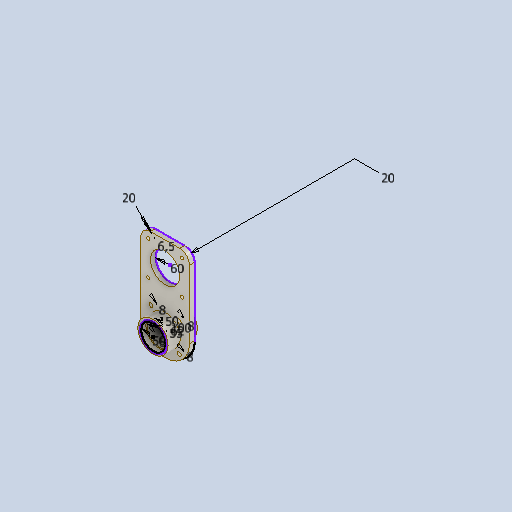
# Autodesk Inventor part: podstwa_obrotowa
Saved by Autodesk Inventor 2023 (Build 270158000, 158)
## iProperties
Created: 2023-03-28
Part Number: podstwa_obrotowa
Material: Tytan
Document SubType Name: Modeling
Designer: krzys
Density: 4.51 g/cm^3
Appearance: Tytan
Mass: 847.85 g
Surface Area: 700.811 cm^2
Volume: 187.993 cm^3
Author: krzys
Autodesk Inventor part; units mm, degrees
ref_plane "YZ Plane" through (0, 0, 0) normal (1, 0, 0) x (0, 1, 0)
ref_plane "XZ Plane" through (0, 0, 0) normal (0, 1, 0) x (-1, 0, 0)
ref_plane "XY Plane" through (0, 0, 0) normal (0, 0, 1) x (1, 0, 0)
sketch "Szkic1" plane through (0, 0, 0) normal (0, 0, 1) x (1, 0, 0)
  circle A0 centre (0, 0) radius 27.5
  circle A1 centre (0, 0) radius 31
  arc A2 (-49.3103, 8.2759) -> (49.3103, 8.2759) centre (0, 0) ccw
  circle A3 centre (0, 110) radius 30
  circle A4 centre (0, 0) radius 25
  circle A5 centre (-28.9914, 28.9914) radius 4
  circle A6 centre (-28.9914, -28.9914) radius 4
  circle A7 centre (28.9914, 28.9914) radius 4
  circle A8 centre (28.9914, -28.9914) radius 4
  circle A9 centre (-34.8003, 144.8003) radius 3.25
  circle A10 centre (-34.8003, 75.1997) radius 3.25
  circle A11 centre (34.8003, 75.1997) radius 3.25
  circle A12 centre (34.8003, 144.8003) radius 3.25
  line L0 (-50, 0) -> (-50, 139.4893)
  line L1 (50, 0) -> (50, 139.4893)
  line L2 (-30, 159.4893) -> (30, 159.4893)
  arc A13 (50, 139.4893) -> (30, 159.4893) centre (30, 139.4893) ccw
  arc A14 (-30, 159.4893) -> (-50, 139.4893) centre (-30, 139.4893) ccw
  dimension "d8" = 360
  dimension "d37" = 360
  dimension "d0" = 55
  dimension "d1" = 62
  dimension "d2" = 100
  dimension "d3" = 60
  dimension "d10" = 50
  dimension "d26" = 8
  dimension "d27" = 8
  dimension "d28" = 8
  dimension "d29" = 8
  dimension "d34" = 6.5
  dimension "d41" = 20
  dimension "d42" = 20
  constraints: 15 centre point, 8 point on circle, 6 end point, 4 coincident, 4 tangent, 1 horizontal, 1 parallel, 1 vertical, 1 other
  measures "d0" diameter of A0
  measures "d1" diameter of A1
  measures "d2" diameter of A2
  measures "d3" diameter of A3
  measures "d10" diameter of A4
  measures "d26" diameter of A5
  measures "d27" diameter of A6
  measures "d28" diameter of A7
  measures "d29" diameter of A8
  measures "d34" diameter of A9
  measures "d41" radius of A13
  measures "d42" radius of A14
extrude "Wyciągnięcie proste1" add sketch "Szkic1" along normal blind 35 contours A1
sketch "Szkic2" plane through (0, 0, 35) normal (0, 0, 1) x (1, 0, 0)
  circle A0 centre (0, 0) radius 25
  circle A1 centre (0, 0) radius 27.4549
  dimension "d15" = 50
  constraints: 2 centre point, 1 coincident
  measures "d15" diameter of A0
extrude "Wyciągnięcie proste3" add sketch "Szkic2" against normal blind 48
extrude "Wyciągnięcie proste5" cut sketch "Szkic2" against normal blind 13
extrude "Wyciągnięcie proste6" add sketch "Szkic1" against normal blind 25 contours A1
extrude "Wyciągnięcie proste7" add sketch "Szkic1" along normal blind 10 contours L0 A14 L2 A13 L1 A2
